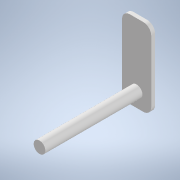
# Autodesk Inventor part: uchwyt_okno
Saved by Autodesk Inventor 2021 (Build 250183000, 183)
## iProperties
Created: 2021-06-22
Part Number: uchwyt_okno
Material: Ogólny
Document SubType Name: Modeling
Designer: Wojciech Wołczek
Density: 1 g/cm^3
Appearance: Domyślna
Author: Wojciech Wołczek
Autodesk Inventor part; units mm, degrees
ref_plane "YZ Plane" through (0, 0, 0) normal (1, 0, 0) x (0, 1, 0)
ref_plane "XZ Plane" through (0, 0, 0) normal (0, 1, 0) x (-1, 0, 0)
ref_plane "XY Plane" through (0, 0, 0) normal (0, 0, 1) x (1, 0, 0)
sketch "Szkic1" plane through (0, 0, 0) normal (0, 0, 1) x (1, 0, 0)
  circle A0 centre (0, 0) radius 3
  dimension "d0" = 6
  constraints: 1 centre point, 1 coincident
  measures "d0" diameter of A0
extrude "Wyciągnięcie proste1" add sketch "Szkic1" along normal blind 50
sketch "Szkic2" plane through (0, 0, 0) normal (0, 0, -1) x (-1, 0, 0)
  line L0 (-7.5, 32.5) -> (7.5, 32.5)
  line L1 (7.5, 32.5) -> (7.5, -7.5)
  line L2 (7.5, -7.5) -> (-7.5, -7.5)
  line L3 (-7.5, -7.5) -> (-7.5, 32.5)
  line L4 (-7.5, 32.5) -> (7.5, -7.5) construction
  line L5 (7.5, 32.5) -> (-7.5, -7.5) construction
  point P0 (0, 0)
  point P1 (0, 12.5)
  dimension "d3" = 40
  dimension "d4" = 15
  dimension "d5" = 7.5
  dimension "d6" = 7.5
  constraints: 12 end point, 2 midpoint, 2 parallel, 1 horizontal, 1 perpendicular
  measures "d3" distance of L0.end L1.end
  measures "d4" distance of L1.end L2.end
  measures "d5" distance from line of point (0, 0) L1
  measures "d6" distance from line of point (0, 0) L2
extrude "Wyciągnięcie proste2" add sketch "Szkic2" along normal blind 2
fillet "Zaokrąglenie1" radius 4 4 edges at (7.5, 32.5, -1) (-7.5, 32.5, -1) (-7.5, -7.5, -1) (7.5, -7.5, -1)
